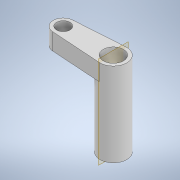
# Autodesk Inventor part: trục quay
Saved by Autodesk Inventor 2020 (Build 240168000, 168)
## iProperties
Created: 2022-11-23
Part Number: trục quay
Material: Generic
Document SubType Name: Modeling
Designer: ADMIN
Density: 1 g/cm^3
Appearance: Default
Author: ADMIN
Autodesk Inventor part; units mm, degrees
ref_plane "XZ Plane" through (0, 0, 0) normal (0, 1, 0) x (-1, 0, 0)
ref_plane "XY Plane" through (0, 0, 0) normal (0, 0, 1) x (1, 0, 0)
sketch "Sketch1" plane through (0, 0, 0) normal (0, 1, 0) x (-1, 0, 0)
  circle A0 centre (0, 0) radius 4
  dimension "d0" = 8
  constraints: 1 centre point, 1 coincident
  measures "d0" diameter of A0
extrude "Extrusion1" add sketch "Sketch1" along normal blind 25
sketch "Sketch2" plane through (0, 25, 0) normal (0, 1, 0) x (1, 0, 0)
  circle A0 centre (0, 0) radius 3
  dimension "d3" = 6
  constraints: 1 centre point, 1 coincident
  measures "d3" diameter of A0
extrude "Extrusion2" cut sketch "Sketch2" against normal blind 13
sketch "Sketch3" plane through (0, 0, 0) normal (1, 0, 0) x (0, 1, 0)
  line L0 (25, -4) -> (25, 4) projected
  circle A0 centre (4, 0) radius 2
  line L1 (0, -4) -> (0, 4) projected
  point P0 (0, 0)
  dimension "d8" = 4
  dimension "d9" = 4
  constraints: 1 centre point
  measures "d8" diameter of A0
  measures "d9" distance from line of L1 A0.centre
extrude "Extrusion3" cut sketch "Sketch3" against normal blind 25
sketch "Sketch4" plane through (0, 25, 0) normal (0, 1, 0) x (1, 0, 0)
  arc A0 (-14.9593, 3.0022) -> (-15.0991, -2.9945) centre (-14.9593, 0.0022) ccw
  circle A1 centre (0, 0) radius 4 projected
  circle A2 centre (0, 0) radius 4 projected
  arc A3 (-0.2686, 3.991) -> (-0.2682, -3.991) centre (0, 0) ccw
  line L0 (-14.9593, 3.0022) -> (-0.2686, 3.991)
  line L1 (-15.0991, -2.9945) -> (-0.2682, -3.991)
  dimension "d12" = 6
  constraints: 6 point on circle, 6 tangent, 4 end point, 2 centre point
  measures "d12" diameter of A0
extrude "Extrusion4" add sketch "Sketch4" against normal blind 5 contours L0 A1 L1 A0
sketch "Sketch5" plane through (0, 25, 0) normal (0, 1, 0) x (1, 0, 0)
  arc A0 (-14.9593, 3.0022) -> (-15.0991, -2.9945) centre (-14.9593, 0.0022) ccw projected
  circle A1 centre (-14.9593, 0.0022) radius 2
  point P0 (0, 0)
  dimension "d15" = 4
  constraints: 1 centre point, 1 coincident
  measures "d15" diameter of A1
hole "Hole1" at (-14.9593, 25, -0.0022) direction (0, -1, 0) diameter 4 end through all
body "Solid1"
